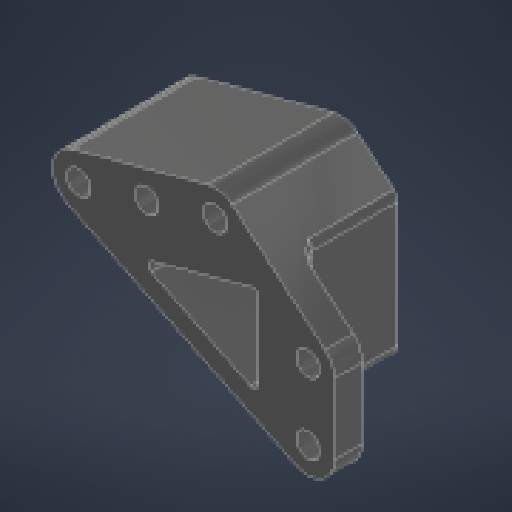
# Autodesk Inventor part: angleblock
Saved by Autodesk Inventor 2025.2 (Build 292293000, 293)
## iProperties
Created: 2025-12-03
Part Number: angleblock
Material: ABS Plastic
Document SubType Name: Modeling
Designer: cloudy
Density: 1.06 g/cm^3
Appearance: Smooth - Dark Gray
Mass: 15.2459 g
Surface Area: 67.1504 cm^2
Volume: 14.3829 cm^3
Author: cloudy
Autodesk Inventor part; units mm, degrees
ref_plane "YZ Plane" through (0, 0, 0) normal (1, 0, 0) x (0, 1, 0)
ref_plane "XZ Plane" through (0, 0, 0) normal (0, 1, 0) x (-1, 0, 0)
ref_plane "XY Plane" through (0, 0, 0) normal (0, 0, 1) x (1, 0, 0)
sketch "Sketch1" plane through (0, 0, 0) normal (0, 0, 1) x (1, 0, 0)
  circle A0 centre (-6.35, 31.75) radius 2.1844 projected
  circle A1 centre (-6.35, 44.45) radius 2.1844 projected
  circle A2 centre (-23.0479, 58.6963) radius 2.1844 projected
  circle A3 centre (-35.2974, 55.3436) radius 2.1844 projected
  circle A4 centre (-47.5468, 51.991) radius 2.1844 projected
  arc A5 (-8.4501, 27.4756) -> (-1.5875, 31.75) centre (-6.35, 31.75) ccw
  arc A6 (-1.5875, 44.45) -> (-3.2589, 48.073) centre (-6.35, 44.45) ccw
  arc A7 (-19.9568, 62.3193) -> (-24.3051, 63.2898) centre (-23.0479, 58.6963) ccw
  arc A8 (-48.8041, 56.5845) -> (-49.647, 47.7165) centre (-47.5468, 51.991) ccw
  line L0 (-49.647, 47.7165) -> (-8.4501, 27.4756)
  line L1 (-1.5875, 31.75) -> (-1.5875, 44.45)
  line L2 (-3.2589, 48.073) -> (-19.9568, 62.3193)
  line L3 (-24.3051, 63.2898) -> (-48.8041, 56.5845)
  point P0 (0, 0)
  dimension "d0" = 9.525
  dimension "d1" = 9.525
  constraints: 8 end point, 8 point on circle, 8 tangent, 4 centre point, 4 coincident, 2 equal radius
  measures "d0" diameter of A5
  measures "d1" diameter of A6
extrude "Extrusion1" add sketch "Sketch1" along normal blind 5.08
sketch "Sketch2" plane through (0, 0, 0) normal (0, 0, -1) x (-1, 0, 0)
  line L0 (12.7, 26.4922) -> (12.7, 87.884) projected
  line L1 (1.5875, 31.75) -> (1.5875, 44.45) projected
  arc A0 (1.5875, 31.75) -> (8.4501, 27.4756) centre (6.35, 31.75) ccw projected
  line L2 (49.647, 47.7165) -> (8.4501, 27.4756) projected
  arc A1 (49.647, 47.7165) -> (48.8041, 56.5845) centre (47.5468, 51.991) ccw projected
  line L3 (24.3051, 63.2898) -> (48.8041, 56.5845) projected
  arc A2 (24.3051, 63.2898) -> (19.9568, 62.3193) centre (23.0479, 58.6963) ccw projected
  line L4 (3.2589, 48.073) -> (19.9568, 62.3193) projected
  arc A3 (3.2589, 48.073) -> (1.5875, 44.45) centre (6.35, 44.45) ccw projected
  circle A4 centre (47.5468, 51.991) radius 2.1844 projected
  circle A5 centre (35.2974, 55.3436) radius 2.1844 projected
  circle A6 centre (23.0479, 58.6963) radius 2.1844 projected
  circle A7 centre (6.35, 44.45) radius 2.1844 projected
  circle A8 centre (6.35, 31.75) radius 2.1844 projected
  point P0 (0, 0)
  point P1 (12.7, 56.128)
  point P2 (12.7, 29.5636)
extrude "Extrusion2" add sketch "Sketch2" along normal blind 17.4625 contours L0 L4 A2 L3 A1 L2
fillet "Fillet1" radius 2 2 edges at (-12.7, 29.5636, -8.7312) (-12.7, 56.128, -8.7312)
fillet "Fillet2" radius 2 3 edges at (-12.8839, 56.0431, 0) (-13.6426, 31.077, 0) (-12.7, 43.99, 0)
sketch "Sketch3" plane through (0, 0, -17.4625) normal (0, 0, -1) x (-1, 0, 0)
  line L0 (36.8861, 45.6918) -> (15.24, 51.6163)
  line L1 (15.24, 51.6163) -> (15.24, 35.0566)
  line L2 (15.24, 35.0566) -> (36.8861, 45.6918)
  line L3 (15.5819, 30.9796) -> (49.647, 47.7165) projected
  line L4 (-20.5952, 64.0577) -> (38.6923, 47.8309) projected
  line L5 (12.7, 26.4922) -> (12.7, 87.884) projected
  point P0 (0, 0)
  dimension "d8" = 3.81
  dimension "d9" = 2.54
  dimension "d10" = 2.54
  constraints: 6 end point, 3 parallel
  measures "d8" distance between parallel lines of L3 L2
  measures "d9" distance between parallel lines of L5 L1
  measures "d10" distance between parallel lines of L4 L0
extrude "Extrusion3" cut sketch "Sketch3" against normal through all
fillet "Fillet3" radius 1 3 edges at (-36.8861, 45.6918, -6.1913) (-15.24, 51.6163, -6.1913) (-15.24, 35.0566, -6.1913)
body "Solid1"
